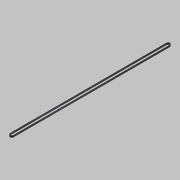
# Autodesk Inventor part: Part18
Saved by Autodesk Inventor 2014 (Build 180170000, 170)
## iProperties
Created: 2016-03-29
Part Number: Part18
Material: Rubber
Document SubType Name: Modeling
Designer: admin
Density: 0.93 g/cm^3
Appearance: Rubber - Black - Version 1.1
Author: admin
Autodesk Inventor part; units mm, degrees
ref_plane "YZ Plane" through (0, 0, 0) normal (1, 0, 0) x (0, 1, 0)
ref_plane "XZ Plane" through (0, 0, 0) normal (0, 1, 0) x (-1, 0, 0)
ref_plane "XY Plane" through (0, 0, 0) normal (0, 0, 1) x (1, 0, 0)
sketch "Sketch1" plane through (0, 0, 0) normal (0, 0, 1) x (1, 0, 0)
  line L0 (0, -573) -> (0, 0) construction
  line L1 (-5.5, -573) -> (-5.5, 0)
  line L2 (5.5, 0) -> (5.5, -573)
  arc A0 (-5.5, -573) -> (5.5, -573) centre (0, -573) ccw
  arc A1 (5.5, 0) -> (-5.5, 0) centre (0, 0) ccw
  line L3 (7, -573) -> (7, 0)
  arc A2 (7, 0) -> (-7, 0) centre (0, 0) ccw
  line L4 (-7, 0) -> (-7, -573)
  arc A3 (-7, -573) -> (7, -573) centre (0, -573) ccw
  circle A4 centre (-0.0376, 0) radius 2.5 projected
  point P0 (0, 0)
  point P1 (0, -286.5)
  dimension "d0" = 1.5
  dimension "d3" = 573
  dimension "d4" = 0
  constraints: 12 end point, 8 point on circle, 4 centre point, 4 tangent, 2 parallel, 1 midpoint, 1 vertical, 3 other
  measures "d0" distance between parallel lines of L2 L3
  measures "d3" distance of point (0, 0) L0.start
  measures "d4" distance of point (0, 0) L0.end
extrude "Extrusion1" add sketch "Sketch1" along normal blind 6 contours A3 L4 A2 L3
body "Solid1"
